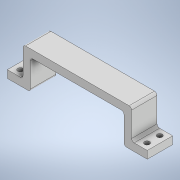
# Autodesk Inventor part: poigne
Saved by Autodesk Inventor 2022 (Build 260153000, 153)
## iProperties
Created: 2022-08-02
Part Number: poigne
Material: Generic
Document SubType Name: Modeling
Designer: thoma
Density: 1 g/cm^3
Appearance: Default
Author: thoma
Autodesk Inventor part; units mm, degrees
ref_plane "YZ Plane" through (0, 0, 0) normal (1, 0, 0) x (0, 1, 0)
ref_plane "XZ Plane" through (0, 0, 0) normal (0, 1, 0) x (-1, 0, 0)
ref_plane "XY Plane" through (0, 0, 0) normal (0, 0, 1) x (1, 0, 0)
sketch "Sketch1" plane through (0, 0, 0) normal (0, 0, 1) x (1, 0, 0)
  line L0 (0, 23.3816) -> (34.8458, 23.3816)
  line L1 (36.8458, 21.3816) -> (36.8458, 2)
  line L2 (38.8458, 0) -> (55.1987, 0)
  line L3 (55.1987, 0) -> (55.1987, 6)
  line L4 (55.1987, 6) -> (44.8458, 6)
  line L5 (42.8458, 8) -> (42.8458, 27.3816)
  line L6 (40.8458, 29.3816) -> (0, 29.3816)
  arc A0 (42.8458, 8) -> (44.8458, 6) centre (44.8458, 8) ccw
  arc A1 (36.8458, 2) -> (38.8458, 0) centre (38.8458, 2) ccw
  arc A2 (36.8458, 21.3816) -> (34.8458, 23.3816) centre (34.8458, 21.3816) ccw
  arc A3 (42.8458, 27.3816) -> (40.8458, 29.3816) centre (40.8458, 27.3816) ccw
  line L7 (0, 23.3816) -> (0, 29.3816)
  point P0 (0, 0)
  dimension "d0" = 6
  dimension "d1" = 6
  dimension "d2" = 6
  dimension "d3" = 2
  constraints: 16 end point, 8 point on circle, 8 tangent, 7 perpendicular, 4 centre point, 3 equal radius, 1 horizontal
  measures "d0" distance between parallel lines of L0 L6
  measures "d1" distance between parallel lines of L1 L5
  measures "d2" distance of L2.end L3.end
  measures "d3" radius of A0
extrude "Extrusion1" add sketch "Sketch1" along normal blind 20
sketch "Sketch2" plane through (44.8458, 6, 0) normal (0, 1, 0) x (1, 0, 0)
  line L0 (10.3529, -20) -> (0, -20) construction
  line L1 (5.1765, -20) -> (5.1765, -15) construction
  line L2 (5.1765, -15) -> (5.1765, -5) construction
  circle A0 centre (5.1765, -15) radius 2
  circle A1 centre (5.1765, -5) radius 2
  point P0 (-44.8458, 0)
  dimension "d7" = 10
  dimension "d8" = 5
  dimension "d9" = 4
  dimension "d10" = 4
  constraints: 4 end point, 2 centre point, 2 coincident, 1 midpoint, 1 point on line, 1 vertical
  measures "d7" distance of L1.end L2.end
  measures "d8" distance of L1.start L1.end
  measures "d9" diameter of A0
  measures "d10" diameter of A1
extrude "Extrusion2" cut sketch "Sketch2" against normal blind 20
mirror "Mirror1" about plane through (0, 29.3816, 0) normal (-1, 0, 0) of "Extrusion1", "Extrusion2"
body "Solid1"
